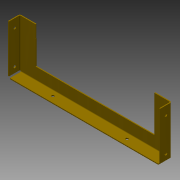
# Autodesk Inventor part: drawer_support
Saved by Autodesk Inventor 2014 SP2 (Build 180246200, 246)
## iProperties
Created: 2016-05-09
Part Number: drawer_support
Material: Generic
Document SubType Name: Sheet Metal
Designer: cruiser
Density: 1 g/cm^3
Sheet Metal Rule: Default_mm
Appearance: Gold
Flat Pattern Width: 10.5991 cm
Flat Pattern Length: 29.1782 cm
Flat Pattern Area: 309.262 cm^2
Sheet Metal Width: 105.991 mm
Sheet Metal Length: 291.782 mm
Sheet Metal Area: 30926.186 mm^2
Author: cruiser
Autodesk Inventor part; units mm, degrees
ref_plane "YZ Plane" through (0, 0, 0) normal (1, 0, 0) x (0, 1, 0)
ref_plane "XZ Plane" through (0, 0, 0) normal (0, 1, 0) x (-1, 0, 0)
ref_plane "XY Plane" through (0, 0, 0) normal (0, 0, 1) x (1, 0, 0)
sketch "Sketch1" plane through (0, 0, 0) normal (0, 1, 0) x (-1, 0, 0)
  line L0 (128.65, -42.7875) -> (-128.65, -42.7875)
  line L1 (-128.65, -42.7875) -> (-128.65, 42.7875)
  line L2 (-128.65, 42.7875) -> (128.65, 42.7875)
  line L3 (128.65, 42.7875) -> (128.65, -42.7875)
  line L4 (128.65, -42.7875) -> (-128.65, 42.7875) construction
  line L5 (-128.65, -42.7875) -> (128.65, 42.7875) construction
  point P0 (0, 0)
  dimension "d0" = 257.3
  dimension "d1" = 85.575
  measures "d0" distance of L1.end L2.end
  measures "d1" distance of L0.end L1.end
extrude "Plate1" add sketch "Sketch1" along normal blind 1.5875
sketch "Sketch2" plane through (-127.0625, 1.5875, -42.7875) normal (-1, 0, 0) x (0, -1, 0)
  line L0 (0, 85.575) -> (0, 0)
  line L1 (0, 0) -> (20, 0)
  line L2 (20, 0) -> (20, 85.575)
  line L3 (20, 85.575) -> (0, 85.575)
  constraints: 6 end point, 1 horizontal, 1 perpendicular, 1 vertical
edge flange "Flange1" height 20 angle 90 thickness 1.5875 bend radius 1.5875 thickness toward (-1, 0, 0) relief straight relief width 1.5875 relief depth 0.7937 corner gap 1.5875 corner form 0 edges at (-128.65, 0, 0) (128.65, 0, 0) wall of the first edge with corners at (-127.0625, 1.5875, 42.7875) (-127.0625, 1.5875, -42.7875) (-127.0625, -18.4125, -42.7875) (-127.0625, -18.4125, 42.7875)
bend "Bend1"
corner "Corner1"
sketch "Sketch3" plane through (0, 1.5875, 0) normal (0, 1, 0) x (1, 0, 0)
  line L0 (-125.475, 42.7875) -> (125.475, 42.7875)
  line L1 (-125.475, 42.7875) -> (125.475, 42.7875)
  line L2 (125.475, 42.7875) -> (125.475, 45.9625)
  line L3 (125.475, 45.9625) -> (-125.475, 45.9625)
  line L4 (-125.475, 45.9625) -> (-125.475, 42.7875)
  line L5 (0, 0) -> (0, 42.7875)
  dimension "d13" = 3.175
  dimension "d14" = 250.95
  measures "d13" distance of L3.end L1.start
  measures "d14" distance of L2.end L3.end
sheet face with bend "Face2" sketch "Sketch3" thickness 1.5875 toward (0, -1, 0) bend radius 1.5875 relief straight relief width 1.5875 relief depth 0.7937
bend "Bend2"
sketch "Sketch21" plane through (0, 1.5875, 0) normal (0, 1, 0) x (1, 0, 0)
  line L0 (-128.65, -42.7875) -> (-100.5, -42.7875)
  line L1 (-100.5, -42.7875) -> (-100.5, -47.7875)
  line L2 (-100.5, -47.7875) -> (-128.65, -47.7875)
  line L3 (-128.65, -47.7875) -> (-128.65, -42.7875)
  line L4 (128.65, -42.7875) -> (-128.65, -42.7875)
  line L5 (0, 0) -> (0, -42.7875)
  dimension "d173" = 100.5
  dimension "d174" = 5
  measures "d173" distance between parallel lines of L5 L1
  measures "d174" distance of L0.end L1.end
sketch "Sketch4" plane through (0, 1.5875, 0) normal (0, 1, 0) x (1, 0, 0)
  line L0 (125.475, 45.9625) -> (-125.475, 45.9625) projected
  line L1 (125.475, -42.7875) -> (-125.475, -42.7875) projected
  line L2 (-100.475, 24.1375) -> (100.475, 24.1375)
  line L3 (100.475, 24.1375) -> (100.475, -42.7875)
  line L4 (100.475, -42.7875) -> (-100.475, -42.7875)
  line L5 (-100.475, -42.7875) -> (-100.475, 24.1375)
  line L6 (0, 0) -> (0, 45.9625)
  line L7 (-125.475, 42.7875) -> (-125.475, -42.7875) projected
  dimension "d21" = 21.825
  dimension "d34" = 25
  constraints: 10 end point, 2 parallel, 1 horizontal, 1 midpoint, 1 perpendicular, 1 point on line, 1 other
  measures "d21" distance between parallel lines of L0 L2
  measures "d34" distance between parallel lines of L7 L5
extrude "Cut1" cut sketch "Sketch4" against normal blind 1.5875
sketch "Sketch19" plane through (0, 1.5875, 0) normal (0, 1, 0) x (1, 0, 0)
  line L0 (-100.475, 24.1375) -> (100.475, 24.1375) projected
  line L1 (-100.475, -42.7875) -> (-100.5, -42.7875)
  line L2 (-100.5, -42.7875) -> (-100.5, -16.1125)
  line L3 (-100.5, -16.1125) -> (-100.475, -16.1125)
  line L4 (-100.475, -16.1125) -> (-100.475, -42.7875)
  line L5 (0, 0) -> (0, 24.1375)
  line L6 (100.475, -42.7875) -> (100.5, -42.7875)
  line L7 (100.5, -42.7875) -> (100.5, -16.1125)
  line L8 (100.5, -16.1125) -> (100.475, -16.1125)
  line L9 (100.475, -16.1125) -> (100.475, -42.7875)
  dimension "d161" = 201
  dimension "d163" = 40.25
  constraints: 18 end point, 3 symmetric about line, 2 parallel, 1 horizontal, 1 midpoint, 1 perpendicular
  measures "d161" distance between parallel lines of L7 L2
  measures "d163" distance between parallel lines of L0 L3
extrude "Cut3" cut sketch "Sketch19" against normal blind 1.5875
sketch "Sketch5" plane through (125.475, 1.5875, -44.375) normal (0, 0, -1) x (-1, 0, 0)
  line L0 (250.95, 0) -> (0, 0)
  line L1 (0, 0) -> (0, -20)
  line L2 (0, -20) -> (250.95, -20)
  line L3 (250.95, -20) -> (250.95, 0)
  constraints: 6 end point, 1 horizontal, 1 perpendicular, 1 vertical
edge flange "Flange2" height 20 angle 90 thickness 1.5875 bend radius 1.5875 thickness toward (0, 0, -1) relief straight relief width 1.5875 relief depth 0.7937 edges at (0, 0, -45.9625) wall of the first edge with corners at (-125.475, 1.5875, -44.375) (125.475, 1.5875, -44.375) (125.475, -18.4125, -44.375) (-125.475, -18.4125, -44.375)
bend "Bend3"
corner "Corner2"
sketch "Sketch16" plane through (118.65, -38.4125, 50.2375) normal (-1, 0, 0) x (0, 0, 1)
  line L0 (0, 36.825) -> (0, 0) projected
  line L1 (-8.4125, 36.825) -> (0, 36.825) projected
  circle A0 centre (-3, 31.825) radius 2.25
  circle A1 centre (-3, 12.825) radius 2.25
  point P0 (-50.2375, 38.4125)
  dimension "d135" = 4.5
  dimension "d136" = 3
  dimension "d137" = 4.5
  dimension "d139" = 3
  dimension "d140" = 19
  dimension "d141" = 5
  constraints: 2 centre point
  measures "d135" diameter of A0
  measures "d136" distance from line of L0 A0.centre
  measures "d137" diameter of A1
  measures "d139" distance from line of L0 A1.centre
  measures "d140" distance of A1.centre A0.centre
  measures "d141" distance from line of L1 A0.centre
cut "Cut2" [suppressed]
sketch "Sketch17" plane through (-128.65, -18.4125, -42.7875) normal (-1, 0, 0) x (0, 0, 1)
  line L0 (85.575, 16.825) -> (0, 16.825)
  line L1 (85.575, 0) -> (160.3375, 0)
  line L2 (160.3375, 0) -> (160.3375, 16.825)
  line L3 (160.3375, 16.825) -> (85.575, 16.825)
  line L4 (85.575, 16.825) -> (85.575, 0)
  point P0 (42.7875, 18.4125)
  point P1 (58.9, 20)
  dimension "d200" = 74.7625
  measures "d200" distance between parallel lines of L4 L2
sketch "Sketch20" plane through (0, 1.5875, 0) normal (0, 1, 0) x (1, 0, 0)
  line L0 (100.5, -42.7875) -> (125.475, -42.7875)
  line L1 (125.475, -42.7875) -> (125.475, -37.0625)
  line L2 (125.475, -37.0625) -> (100.5, -37.0625)
  line L3 (100.5, -37.0625) -> (100.5, -42.7875)
  point P0 (0, 0)
  constraints: 8 end point, 2 parallel, 1 horizontal, 1 perpendicular
cut "Cut4" [suppressed]
sketch "Sketch22" plane through (0, 1.5875, 0) normal (0, 1, 0) x (1, 0, 0)
  line L0 (-100.5, -16.1125) -> (-117, -16.1125)
  line L1 (-117, -16.1125) -> (-117, -42.7875)
  line L2 (-117, -42.7875) -> (-100.5, -42.7875)
  line L3 (-100.5, -42.7875) -> (-100.5, -16.1125)
  line L4 (-100.475, -16.1125) -> (-100.475, 24.1375) projected
  line L5 (-117, -16.1125) -> (-100.475, -16.1125)
  line L6 (-100.475, -16.1125) -> (-100.475, 2.2125)
  line L7 (-100.475, 2.2125) -> (-117, 2.2125)
  line L8 (-117, 2.2125) -> (-117, -16.1125)
  line L9 (-100.5, -42.7875) -> (-125.475, -42.7875) projected
  point P0 (0, 0)
  dimension "d176" = 16.5
  dimension "d196" = 45
  dimension "d199" = 0
  constraints: 16 end point, 4 parallel, 2 horizontal, 2 perpendicular, 1 point on line
  measures "d176" distance of L0.start L0.end
  measures "d196" distance between parallel lines of L7 L2
  measures "d199" distance between parallel lines of L9 L2
cut "Cut5" [suppressed]
sketch "Sketch24" plane through (-117, 13, 40.2375) normal (1, 0, 0) x (0, 0, -1)
  line L0 (0, 0) -> (43.4125, 0) projected
  line L1 (0, -9.825) -> (0, 0) projected
  circle A0 centre (5, -3) radius 2.25
  circle A1 centre (24, -3) radius 2.25
  point P0 (40.2375, -13)
  dimension "d189" = 4.5
  dimension "d190" = 4.5
  dimension "d192" = 3
  dimension "d193" = 3
  dimension "d194" = 19
  dimension "d195" = 5
  constraints: 2 centre point
  measures "d189" diameter of A0
  measures "d190" diameter of A1
  measures "d192" distance from line of L0 A0.centre
  measures "d193" distance from line of L0 A1.centre
  measures "d194" distance of A0.centre A1.centre
  measures "d195" distance from line of L1 A0.centre
cut "Cut6" [suppressed]
sketch "Sketch25" plane through (125.475, -18.4125, -45.9625) normal (0, 0, -1) x (-1, 0, 0)
  line L0 (250.95, 0) -> (0, 0) projected
  circle A0 centre (62.725, 10) radius 2.25
  line L1 (125.475, 18.4125) -> (125.475, 0)
  circle A1 centre (188.225, 10) radius 2.25
  dimension "d201" = 4.5
  dimension "d202" = 62.75
  dimension "d203" = 10
  constraints: 2 centre point, 2 end point, 1 midpoint, 1 symmetric about line, 1 other
  measures "d201" diameter of A0
  measures "d202" distance from line of L1 A0.centre
  measures "d203" distance from line of L0 A0.centre
extrude "Cut7" cut sketch "Sketch25" against normal blind 1.5875
sketch "Sketch26" plane through (128.65, -18.4125, -42.7875) normal (1, 0, 0) x (0, 0, -1)
  line L0 (0, 0) -> (-85.575, 0) projected
  circle A0 centre (-70.5188, 10) radius 2.25
  line L1 (4.7625, 68) -> (-85.575, 68)
  line L2 (-85.575, 68) -> (-85.575, -56.203)
  line L3 (-85.575, -56.203) -> (4.7625, -56.203)
  line L4 (4.7625, -56.203) -> (4.7625, 68)
  line L5 (-85.575, 20) -> (0, 20) projected
  line L6 (3.175, 0) -> (3.175, 16.825) projected
  line L7 (-40.4062, -56.203) -> (-40.4063, 68)
  circle A1 centre (-10.2938, 10) radius 2.25
  point P0 (-77.3, 0)
  point P1 (-42.7875, 18.4125)
  point P2 (-77.3, 40)
  point P3 (0, 20)
  dimension "d206" = 10
  dimension "d207" = 4.5
  dimension "d208" = 90.3375
  dimension "d209" = 48
  dimension "d210" = 1.5875
  dimension "d211" = 30.1125
  constraints: 10 end point, 2 centre point, 2 midpoint, 2 parallel, 1 horizontal, 1 perpendicular, 1 symmetric about line, 2 other
  measures "d206" distance from line of L0 A0.centre
  measures "d207" diameter of A0
  measures "d208" distance of L1.start L1.end
  measures "d210" distance between parallel lines of L6 L4
  measures "d211" distance from line of L7 A0.centre
extrude "Cut8" cut sketch "Sketch26" against normal through all contours A0 | A1
sketch "Sketch14" plane through (128.65, -1.5875, 41.2) normal (0, 0, 1) x (1, 0, 0)
  line L0 (0, -16.825) -> (0, 0)
  line L1 (0, 0) -> (-10, 0)
  line L2 (-10, 0) -> (-10, -16.825)
  line L3 (-10, -16.825) -> (0, -16.825)
  constraints: 6 end point, 1 horizontal, 1 perpendicular, 1 vertical
sketch "Sketch15" plane through (120.2375, -38.4125, 38.65) normal (-1, 0, 0) x (0, -1, 0)
  line L0 (-36.825, 0) -> (0, 0)
  line L1 (0, 0) -> (0, 11.5875)
  line L2 (0, 11.5875) -> (-36.825, 11.5875)
  line L3 (-36.825, 11.5875) -> (-36.825, 0)
  constraints: 6 end point, 1 horizontal, 1 perpendicular, 1 vertical
sketch "Sketch18" plane through (-128.65, -38.4125, 113.4125) normal (0, 0, 1) x (1, 0, 0)
  line L0 (0, 36.825) -> (0, 0)
  line L1 (0, 0) -> (20, 0)
  line L2 (20, 0) -> (20, 36.825)
  line L3 (20, 36.825) -> (0, 36.825)
  constraints: 6 end point, 1 horizontal, 1 perpendicular, 1 vertical
sketch "Sketch23" plane through (-118.5875, 0, -4.7625) normal (1, 0, 0) x (0, 1, 0)
  line L0 (0, 45) -> (0, 1.5875)
  line L1 (0, 1.5875) -> (13, 1.5875)
  line L2 (13, 1.5875) -> (13, 45)
  line L3 (13, 45) -> (0, 45)
  constraints: 8 end point
equation "\"d0\" = drawer_x"
equation "\"d1\" = drawer_y - 3 * sm_thickness"
equation "\"d13\" = 2 * sm_thickness"
equation "\"d14\" = drawer_x - 4 * sm_thickness"
equation "\"d22\" = Thickness"
equation "\"d142\" = Thickness"
equation "\"Thickness\" = sm_thickness"
equation "\"d3\" = BendReliefWidth"
equation "\"d4\" = BendReliefDepth"
equation "\"d5\" = MinimumRemnant"
equation "\"d6\" = BendRadius"
equation "\"d7\" = drawer_support_overlap"
equation "\"d9\" = BendRadius"
equation "\"d10\" = CornerReliefSize"
equation "\"d11\" = GapSize"
equation "\"d12\" = JacobiRadiusSize"
equation "\"d15\" = BendRadius"
equation "\"d16\" = BendReliefWidth"
equation "\"d18\" = MinimumRemnant"
equation "\"d17\" = BendReliefDepth"
equation "\"d19\" = BendRadius"
equation "\"d24\" = BendReliefWidth"
equation "\"d25\" = BendReliefDepth"
equation "\"d26\" = MinimumRemnant"
equation "\"d27\" = BendRadius"
equation "\"d28\" = drawer_support_overlap"
equation "\"d30\" = BendRadius"
equation "\"d31\" = CornerReliefSize"
equation "\"d32\" = GapSize"
equation "\"d33\" = JacobiRadiusSize"
equation "\"BendRadius\" = Thickness"
equation "\"BendReliefWidth\" = Thickness"
equation "\"BendReliefDepth\" = 0.5 * Thickness"
equation "\"CornerReliefSize\" = 4 * Thickness"
equation "\"MinimumRemnant\" = 2 * Thickness"
equation "\"TransitionRadius\" = BendRadius"
equation "\"JacobiRadiusSize\" = BendRadius"
equation "\"GapSize\" = Thickness"
equation "\"sm_thickness\" = 1.5875"
equation "\"very_thick_acrylic\" = 9.45"
equation "\"thick_acrylic\" = 5.88"
equation "\"thin_acrylic\" = 3.15"
equation "\"clear_acrylic\" = 3.15"
equation "\"wood_thickness\" = 6.72"
equation "\"m3_diameter\" = 3"
equation "\"m3_head\" = 6"
equation "\"m4_diameter\" = 4"
equation "\"m5_diameter\" = 5"
equation "\"m5_head\" = 10.3"
equation "\"brass_insert_drill\" = 4"
equation "\"m5_brass_insert_drill\" = 6.7"
equation "\"m3_press_nut_drill\" = 4.5"
equation "\"m5_press_nut_drill\" = 6.5"
equation "\"stepper_screw_space\" = 35"
equation "\"stepper_shaft_diameter\" = 5"
equation "\"stepper_body_diameter\" = 28"
equation "\"laser_body_diameter\" = 12"
equation "\"carrier_y\" = 251"
equation "\"carrier_z\" = 12"
equation "\"visor_x\" = 253.925"
equation "\"visor_y\" = 85.6"
equation "\"window_z\" = 332.225"
equation "\"window_y\" = 93.75"
equation "\"window_overlap\" = 48"
equation "\"acrylic_into_frame\" = 5"
equation "\"door_x\" = 251"
equation "\"door_z\" = 332.225"
equation "\"door_overlap\" = 48"
equation "\"reservoir_x\" = 201"
equation "\"reservoir_y\" = 201"
equation "\"linear_bearing_spacing\" = 271"
equation "\"tray_border\" = 25"
equation "\"tray_x\" = 251"
equation "\"tray_y\" = 251"
equation "\"bed_z\" = 25"
equation "\"crane_z2\" = 12"
equation "\"end_stop_spacing\" = 19"
equation "\"thumb_nut_offset_y\" = 0"
equation "\"thumb_nut_diameter\" = 7"
equation "\"z_min_from_center\" = 115"
equation "\"frame_top_z\" = 385"
equation "\"frame_bottom_z\" = 275"
equation "\"frame_total_z\" = 661.5875"
equation "\"frame_border\" = 48.0375"
equation "\"frame_foot_z\" = 12"
equation "\"frame_tilt\" = 1deg"
equation "\"subframe_x\" = 66"
equation "\"subframe_y_offset\" = 27.5"
equation "\"laser_y_offset\" = 19.4"
equation "\"laser_diameter\" = 12"
equation "\"laser_z_offset\" = 55"
equation "\"laser_y\" = 15"
equation "\"laser_z\" = 75"
equation "\"t_galvo_frame\" = 6.72"
equation "\"galvo_frame_x\" = 66"
equation "\"galvo_frame_z\" = 65"
equation "\"galvo_frame_y_offset\" = 27.5"
equation "\"drawer_x\" = 257.3"
equation "\"drawer_y\" = 90.3375"
equation "\"drawer_z\" = 278.175"
equation "\"drawer_z_from_bottom\" = 25"
equation "\"nema17_x\" = 43"
equation "\"d2\" = BendRadius"
equation "\"drawer_support_from_top\" = 48"
equation "\"d138\" = 3"
equation "\"d191\" = 3"
equation "\"laser_gap\" = 1"
equation "\"frame_screw_from_center\" = 25"
equation "\"drawer_screw_from_center\" = 55"
equation "\"frame_face_y\" = 45"
equation "\"switch_spacing\" = 19"
equation "\"subframe_y\" = 55"
equation "\"al_thickness\" = 1.5875"
equation "\"rivet_diameter\" = 3.3"
equation "\"bend_factor\" = 2.26205"
equation "\"sm_bend\" = 3.591"
equation "\"al_bend\" = 3.591"
equation "\"frame_x\" = 353.375"
equation "\"carrier_z2\" = 25"
equation "\"carrier_y2\" = 76.825"
equation "\"drawer_support_overlap\" = 20"
body "Solid1"
